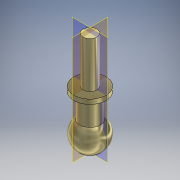
# Autodesk Inventor part: joint_ball_upper
Saved by Autodesk Inventor 2017 (Build 210142000, 142)
## iProperties
Created: 2017-04-26
Part Number: joint_ball_upper
Material: Mosiądz, miękki żółty
Document SubType Name: Modeling
Designer: Speed King
Density: 8.47 g/cm^3
Appearance: Złoty — metal
Mass: 2.689 g
Surface Area: 3.34716 cm^2
Volume: 0.317474 cm^3
Author: Speed King
Autodesk Inventor part; units mm, degrees
sketch "Szkic1" plane through (0, 0, 0) normal (0, 0, 1) x (1, 0, 0)
  arc A0 (0, -3.5) -> (0, 3.5) centre (0, 0) ccw
  line L0 (0, 3.5) -> (0, -3.5)
  line L1 (-0.7, 0) -> (4.2, 0) projected
  line L2 (0, 4.9) -> (0, -4.9) projected
  dimension "d0" = 7
  constraints: 2 end point, 2 point on circle, 2 point on line, 1 centre point, 1 coincident, 1 collinear, 1 vertical
  measures "d0" diameter of A0
revolve "Obrót1" add sketch "Szkic1" angle 360 about axis through (0, 0, 0) along (0, -1, 0)
ref_plane "Płaszczyzna konstrukcyjna1" through (0, 0, 2.65) normal (0, 0, 1) x (1, 0, 0)
sketch "Szkic2" plane through (0, 0, 0) normal (1, 0, 0) x (0, 1, 0)
  line L0 (-5.1683, 2.65) -> (4.9447, 2.65) projected
  line L1 (3.5, 2.65) -> (-3.7236, 2.65)
  line L2 (-3.7236, 2.65) -> (-3.7236, 4.235)
  line L3 (-3.7236, 4.235) -> (3.5, 4.235)
  line L4 (3.5, 4.235) -> (3.5, 2.65)
  point P0 (0, 0)
  constraints: 8 end point, 2 parallel, 1 horizontal, 1 perpendicular, 1 point on line
extrude "Wyciągnięcie proste1" cut sketch "Szkic2" along normal mid plane 10
mirror "Odbij1" about plane through (0, 0, 0) normal (0, 0, 1) of "Wyciągnięcie proste1"
sketch "Szkic3" plane through (0, 0, 2.65) normal (0, 0, 1) x (1, 0, 0)
  circle A0 centre (0, 0) radius 2.2864 projected
extrude "Wyciągnięcie proste2" add sketch "Szkic3" along normal blind 4.5
sketch "Szkic4" plane through (0, 0, 7.15) normal (0, 0, 1) x (1, 0, 0)
  circle A0 centre (0, 0) radius 2.2864 projected
  point P0 (0, 0)
ref_plane "Płaszczyzna konstrukcyjna2" through (0, 0, 7.85) normal (0, 0, 1) x (1, 0, 0)
sketch "Szkic5" plane through (0, 0, 7.85) normal (0, 0, 1) x (1, 0, 0)
  circle A0 centre (0, 0) radius 3.5
  point P0 (0, 0)
  dimension "d8" = 7
  constraints: 1 centre point, 1 coincident
  measures "d8" diameter of A0
loft "Wyciągnięcie złożone1" add profiles "Szkic5" section 1 edges at (-2.2864, 0, 7.15)
sketch "Szkic6" plane through (0, 0, 7.85) normal (0, 0, 1) x (1, 0, 0)
  circle A0 centre (0, 0) radius 3.5 projected
extrude "Wyciągnięcie proste3" add sketch "Szkic6" along normal blind 1
sketch "Szkic7" plane through (0, 0, 8.85) normal (0, 0, 1) x (1, 0, 0)
  circle A0 centre (0, 0) radius 1.5
  point P0 (0, 0)
  dimension "d15" = 3
  constraints: 1 centre point, 1 coincident
  measures "d15" diameter of A0
extrude "Wyciągnięcie proste4" add sketch "Szkic7" along normal blind 10
